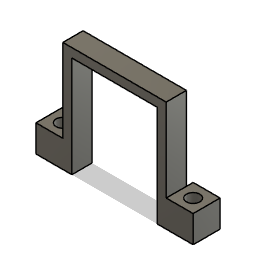
Fixation moto-réducteur (Autodesk Fusion 360 design; units mm, degrees)
Autodesk Fusion 360 part; units mm, degrees
sketch "Sketch1" plane through (0, 0, 0) normal (0, 0, 1) x (1, 0, 0)
  line L0 (0, 0) -> (6, 0)
  line L1 (6, 0) -> (6, 6)
  line L2 (6, 6) -> (0, 6)
  line L3 (0, 6) -> (0, 0)
  line L4 (6, 0) -> (8, 0)
  line L5 (8, 0) -> (8, 24.5)
  line L6 (8, 24.5) -> (6, 24.5)
  line L7 (6, 24.5) -> (6, 0)
  line L8 (6, 24.5) -> (17.5, 24.5)
  line L9 (17.5, 24.5) -> (17.5, 22.5)
  line L10 (17.5, 22.5) -> (6, 22.5)
  line L11 (6, 22.5) -> (6, 24.5)
  line L12 (29, 6) -> (35, 6)
  line L13 (17.5, 22.5) -> (29, 22.5)
  line L14 (29, 0) -> (29, 6)
  line L15 (35, 6) -> (35, 0)
  line L16 (29, 24.5) -> (29, 0)
  line L17 (27, 24.5) -> (29, 24.5)
  line L18 (17.5, 24.5) -> (17.5, 22.5)
  line L19 (29, 22.5) -> (29, 24.5)
  line L20 (35, 0) -> (29, 0)
  line L21 (29, 24.5) -> (17.5, 24.5)
  line L22 (27, 0) -> (27, 24.5)
  line L23 (29, 0) -> (27, 0)
  point P0 (35, 0)
  dimension "d1" = 6
  dimension "d2" = 6
  dimension "d3" = 2
  dimension "d4" = 24.5
  dimension "d5" = 11.5
  dimension "d6" = 2
  constraint horizontal L0
  constraint vertical L1
  constraint horizontal L2
  constraint vertical L3
  constraint coincident L0.start L3.end
  constraint horizontal L4
  constraint vertical L5
  constraint horizontal L6
  constraint vertical L7
  constraint horizontal L8
  constraint vertical L9
  constraint horizontal L10
  constraint vertical L11
  constraint symmetric L0.start L9 L15.end
  constraint symmetric L0.start L9 P0
  constraint symmetric L0.end L9 L14.start
  constraint symmetric L1.end L9 L12.start
  constraint symmetric L2.end L9 L12.end
  constraint symmetric L4.end L9 L22.start
  constraint symmetric L5.end L9 L17.start
  constraint symmetric L6.end L9 L16.start
  constraint symmetric L8.end L9 L18.start
  constraint symmetric L10.start L9 L13.start
  constraint symmetric L10.end L9 L13.end
  measures "d1" distance of L0.start L0.end
  measures "d2" distance of L0.start L2.end
  measures "d3" distance of L0.end L4.end
  measures "d4" distance of L0.end L6.end
  measures "d5" distance of L6.end L8.end
  measures "d6" distance of L6.end L10.end
extrude "Extrude1" add sketch "Sketch1" along normal blind 3 and the other way blind 3 contours L0 L1 L2 L3 L7 | L12 L14 L15 L16 L20 makes body 1 at (31, 6, -1) makes body 2 at (0, 2, 1)
extrude "Extrude2" add sketch "Sketch1" along normal blind 1.5 and the other way blind 1.5 contours L1 L4 L5 L7 L10 | L5 L6 L7 L8 L10 L11 | L5 L8 L9 L10 L18 | L9 L13 L18 L21 L22 | L13 L16 L17 L19 L21 L22 | L13 L14 L16 L22 L23 bodies 1 2
sketch "Sketch3" plane through (0, 6, 0) normal (0, 1, 0) x (-1, 0, 0)
  line L0 (0, -3) -> (0, 3)
  line L1 (0, 3) -> (-6, 3)
  line L2 (-6, 3) -> (-6, 1.5)
  line L3 (-6, 1.5) -> (-6, -1.5)
  line L4 (-6, -1.5) -> (-6, -3)
  line L5 (-6, -3) -> (0, -3)
  circle A0 centre (-3, 0) radius 1.5
  circle A1 centre (-32, 0) radius 1.5
  line L6 (-35, -3) -> (-35, 3)
  line L7 (-29, -3) -> (-35, -3)
  dimension "d16" = 3
  dimension "d17" = 3
  dimension "d18" = 3
  dimension "d19" = 3
  dimension "d20" = 3
  dimension "d21" = 3
  measures "d16" diameter of A0
  measures "d17" diameter of A1
  measures "d18" distance of L5 A0.centre
  measures "d19" distance of L0 A0.centre
  measures "d20" distance of A1.centre L6
  measures "d21" distance of A1.centre L7
extrude "Extrude3" cut sketch "Sketch3" against normal blind 11 contours A0 | A1 bodies 1
extrude "Extrude4" add 1 faces at (27.6667, 9.5, 1.5) along direction (0, 0, 1) up to surface (1.5 mm away) on bodies 1 bodies 1
